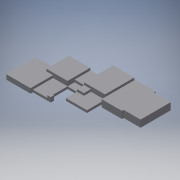
# Autodesk Inventor part: Sportcenter
Saved by Autodesk Inventor 2018.3 (Build 223284000, 284)
## iProperties
Created: 2020-12-08
Part Number: Sportcenter
Material: Generic
Document SubType Name: Modeling
Designer: daanv
Density: 1 g/cm^3
Appearance: Default
Author: daanv
Autodesk Inventor part; units mm, degrees
ref_plane "YZ Plane" through (0, 0, 0) normal (1, 0, 0) x (0, 1, 0)
ref_plane "XZ Plane" through (0, 0, 0) normal (0, 1, 0) x (-1, 0, 0)
ref_plane "XY Plane" through (0, 0, 0) normal (0, 0, 1) x (1, 0, 0)
sketch "Sketch1" plane through (0, 0, 0) normal (0, 0, 1) x (1, 0, 0)
  line L0 (0, 0) -> (49.58, 0)
  line L1 (49.58, 0) -> (49.58, 44.9)
  line L2 (49.58, 44.9) -> (0, 44.9)
  line L3 (0, 44.9) -> (0, 0)
  line L4 (49.58, 2.33) -> (27.13, 2.33)
  line L5 (27.13, 2.33) -> (27.13, 0)
  line L6 (27.13, 44.9) -> (27.13, 42.57)
  line L7 (27.13, 42.57) -> (49.58, 42.57)
  dimension "d0" = 49.58
  dimension "d1" = 44.9
  dimension "d2" = 22.45
  dimension "d3" = 2.33
  constraints: 16 end point, 6 point on line, 3 parallel, 3 perpendicular, 1 horizontal
  measures "d0" distance of L2.end L1.end
  measures "d1" distance of L1.end L0.end
  measures "d2" distance of L4.start L4.end
  measures "d3" distance of L6.start L6.end
extrude "Extrusion1" add sketch "Sketch1" along normal blind 9.35 contours L3 L2 L6 L7 L1 L4 L5 L0
sketch "Sketch2" plane through (0, 0, 0) normal (-1, 0, 0) x (0, 0, 1)
  line L0 (0, 44.9) -> (0, 0) projected
  line L1 (9.35, 44.9) -> (9.35, 0) projected
  line L2 (0, 44.9) -> (9.35, 44.9) projected
  line L3 (0, 39.74) -> (9.35, 39.74)
  line L4 (9.35, 39.74) -> (9.35, 7.69)
  line L5 (9.35, 7.69) -> (0, 7.69)
  line L6 (0, 7.69) -> (0, 39.74)
  dimension "d6" = 32.05
  dimension "d7" = 5.16
  constraints: 8 end point, 2 parallel, 2 point on line, 1 horizontal, 1 perpendicular
  measures "d6" distance of L3.end L4.end
  measures "d7" distance between parallel lines of L2 L3
extrude "Extrusion2" add sketch "Sketch2" along normal blind 31.18 contours L3 L1 L5 L0
sketch "Sketch3" plane through (0, 0, 9.35) normal (0, 0, 1) x (1, 0, 0)
  line L0 (0, 39.74) -> (-31.18, 39.74) projected
  line L1 (-3.12, 39.74) -> (0, 39.74)
  line L2 (0, 39.74) -> (0, 7.69)
  line L3 (0, 7.69) -> (-3.12, 7.69)
  line L4 (-3.12, 7.69) -> (-3.12, 39.74)
  constraints: 8 end point, 2 parallel, 1 horizontal, 1 perpendicular, 1 point on line
extrude "Extrusion3" cut sketch "Sketch3" against normal blind 3.12
sketch "Sketch4" plane through (-31.18, 39.74, 0) normal (0, 1, 0) x (1, 0, 0)
  line L0 (0, -9.35) -> (0, 0) projected
  line L1 (28.06, -9.35) -> (0, -9.35) projected
  line L2 (31.18, 0) -> (0, 0) projected
  line L3 (28.06, -9.35) -> (0, -9.35)
  line L4 (0, -9.35) -> (0, 0)
  line L5 (0, 0) -> (28.06, 0)
  line L6 (28.06, 0) -> (28.06, -9.35)
  constraints: 8 end point, 2 parallel, 1 horizontal, 1 perpendicular
extrude "Extrusion4" add sketch "Sketch4" along normal blind 6.86
sketch "Sketch5" plane through (-31.18, 7.69, 0) normal (0, -1, 0) x (1, 0, 0)
  line L0 (28.06, 0) -> (0, 0) projected
  line L1 (28.06, 9.35) -> (28.06, 0) projected
  line L2 (0, 0) -> (28.06, 0)
  line L3 (28.06, 0) -> (28.06, 3.12)
  line L4 (28.06, 3.12) -> (0, 3.12)
  line L5 (0, 3.12) -> (0, 0)
  dimension "d14" = 3.12
  constraints: 8 end point, 2 parallel, 1 horizontal, 1 perpendicular, 1 point on line
  measures "d14" distance of L3.end L2.end
extrude "Extrusion5" add sketch "Sketch5" along normal blind 24.01
sketch "Sketch6" plane through (-31.18, 7.69, 3.12) normal (0, 0, 1) x (1, 0, 0)
  line L0 (0, 0) -> (9.35, 0)
  line L1 (9.35, 0) -> (9.35, -9.35)
  line L2 (9.35, -9.35) -> (0, -9.35)
  line L3 (0, -9.35) -> (0, 0)
  point P0 (31.18, -7.69)
  dimension "d17" = 9.35
  dimension "d18" = 9.35
  constraints: 8 end point, 2 parallel, 1 horizontal, 1 perpendicular
  measures "d17" distance of L1.end L2.end
  measures "d18" distance of L0.end L1.end
extrude "Extrusion6" add sketch "Sketch6" along normal blind 3.12
sketch "Sketch7" plane through (-31.18, 0, 0) normal (-1, 0, 0) x (0, 0, 1)
  line L0 (3.12, 7.69) -> (0, 7.69) projected
  line L1 (3.12, -1.66) -> (0, -1.66)
  line L2 (0, -1.66) -> (0, 7.69)
  line L3 (0, 7.69) -> (3.12, 7.69)
  line L4 (3.12, 7.69) -> (3.12, -1.66)
  line L5 (0, 7.69) -> (6.24, 7.69)
  line L6 (6.24, 7.69) -> (6.24, 35.13)
  line L7 (6.24, 35.13) -> (0, 35.13)
  line L8 (0, 35.13) -> (0, 7.69)
  line L9 (0, -16.32) -> (0, 46.6) projected
  point P0 (0, 0)
  dimension "d21" = 27.44
  dimension "d24" = 6.24
  constraints: 16 end point, 4 parallel, 2 horizontal, 2 perpendicular
  measures "d21" distance of L6.end L5.end
  measures "d24" distance between parallel lines of L9 L6
extrude "Extrusion7" add sketch "Sketch7" along normal blind 12.47
sketch "Sketch8" plane through (-31.18, 35.13, 6.24) normal (0, 1, 0) x (1, 0, 0)
  line L0 (-12.47, 0) -> (-12.47, 6.24) projected
  line L1 (0, 6.24) -> (-12.47, 6.24) projected
  line L2 (0, 0) -> (-12.47, 0) projected
  line L3 (0, 6.24) -> (-3.12, 6.24)
  line L4 (-3.12, 6.24) -> (-3.12, 0)
  line L5 (-3.12, 0) -> (0, 0)
  line L6 (0, 0) -> (0, 6.24)
  point P0 (31.18, 6.24)
  dimension "d25" = 3.12
  constraints: 8 end point, 2 parallel, 1 horizontal, 1 perpendicular, 1 point on line
  measures "d25" distance of L5.end L4.end
extrude "Extrusion8" cut sketch "Sketch8" against normal blind 6.24 contours L0 L1 L4 L2
sketch "Sketch9" plane through (-43.65, 0, 0) normal (-1, 0, 0) x (0, 0, 1)
  line L0 (0, 28.89) -> (0, -1.66) projected
  line L1 (0, 28.58) -> (9.35, 28.58)
  line L2 (9.35, 28.58) -> (9.35, -1.66)
  line L3 (9.35, -1.66) -> (0, -1.66)
  line L4 (0, -1.66) -> (0, 28.58)
  point P0 (0, 0)
  constraints: 8 end point, 2 parallel, 1 horizontal, 1 perpendicular, 1 point on line
extrude "Extrusion9" add sketch "Sketch9" along normal blind 28.06
sketch "Sketch10" plane through (-71.71, 0, 0) normal (-1, 0, 0) x (0, 0, 1)
  line L0 (0, 28.58) -> (0, -1.66) projected
  line L1 (0, 7.69) -> (6.24, 7.69)
  line L2 (6.24, 7.69) -> (6.24, -31.6)
  line L3 (6.24, -31.6) -> (0, -31.6)
  line L4 (0, -31.6) -> (0, 7.69)
  point P0 (0, 0)
  dimension "d30" = 39.29
  constraints: 8 end point, 2 parallel, 1 horizontal, 1 perpendicular, 1 point on line
  measures "d30" distance of L1.end L2.end
extrude "Extrusion10" add sketch "Sketch10" along normal blind 23.7
sketch "Sketch11" plane through (-71.71, 0, 0) normal (1, 0, 0) x (0, 0, -1)
  line L0 (0, -1.66) -> (-6.24, -1.66) projected
  line L1 (-6.24, -1.66) -> (-6.24, -31.6) projected
  line L2 (-6.24, -31.6) -> (0, -31.6) projected
  line L3 (0, -31.6) -> (0, -1.66) projected
  point P0 (0, 0)
extrude "Extrusion11" add sketch "Sketch11" along normal blind 8.73
sketch "Sketch12" plane through (-62.98, 0, 0) normal (1, 0, 0) x (0, 0, -1)
  line L0 (0, -1.66) -> (-3.12, -1.66)
  line L1 (-3.12, -1.66) -> (-3.12, -28.48)
  line L2 (-3.12, -28.48) -> (0, -28.48)
  line L3 (0, -28.48) -> (0, -1.66)
  point P0 (0, 0)
  dimension "d35" = 26.82
  constraints: 8 end point, 2 parallel, 1 horizontal, 1 perpendicular
  measures "d35" distance of L1.end L0.end
extrude "Extrusion12" add sketch "Sketch12" along normal blind 19.33
sketch "Sketch13" plane through (-43.65, 0, 0) normal (1, 0, 0) x (0, 0, -1)
  line L0 (0, -28.48) -> (-6.24, -28.48)
  line L1 (-6.24, -28.48) -> (-6.24, -24.11)
  line L2 (-6.24, -24.11) -> (0, -24.11)
  line L3 (0, -24.11) -> (0, -28.48)
  point P0 (0, 0)
  dimension "d38" = 6.24
  dimension "d39" = 4.37
  constraints: 8 end point, 2 parallel, 1 horizontal, 1 perpendicular
  measures "d38" distance of L1.end L2.end
  measures "d39" distance of L0.end L1.end
extrude "Extrusion13" add sketch "Sketch13" along normal blind 4.37
body "Solid1"
